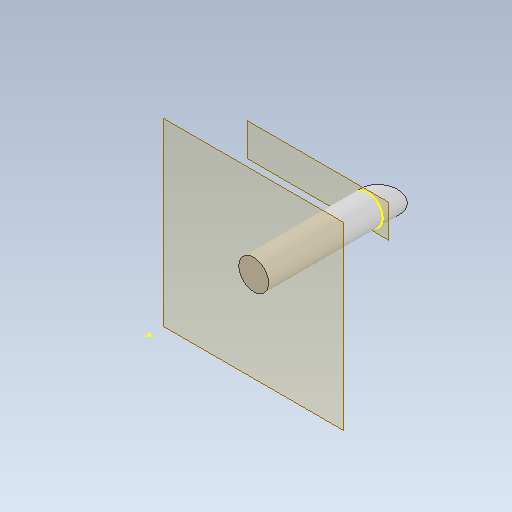
# Autodesk Inventor part: notch piston
Saved by Autodesk Inventor 2021 (Build 250183000, 183)
## iProperties
Created: 2021-03-12
Part Number: notch piston
Material: Generic
Document SubType Name: Modeling
Designer: teh18
Density: 1 g/cm^3
Appearance: Default
Author: teh18
Autodesk Inventor part; units mm, degrees
ref_plane "YZ Plane" through (0, 0, 0) normal (1, 0, 0) x (0, 1, 0)
ref_plane "XZ Plane" through (0, 0, 0) normal (0, 1, 0) x (-1, 0, 0)
sketch "Sketch1" plane through (0, 0, 0) normal (0, 0, 1) x (1, 0, 0)
  point P0 (0, 0)
ref_plane "Work Plane1" through (0, 0, -35) normal (0, 0, 1) x (1, 0, 0)
sketch "Sketch2" plane through (0, 0, -35) normal (0, 0, 1) x (1, 0, 0)
  circle A0 centre (0, 0) radius 5
  dimension "d0" = 10
  constraints: 1 centre point, 1 coincident
  measures "d0" diameter of A0
ref_plane "Work Plane2" through (46.1021, -24.8658, -116.0377) normal (0.6428, 0, 0.766) x (0.766, 0, -0.6428)
extrude "Extrusion1" add sketch "Sketch2" against normal up to surface surface through (46.1021, -24.8658, -116.0377) normal (0.6428, 0, 0.766)
ref_plane "Work Plane3" through (-5, 0, -73.1579) normal (0, 0, 1) x (1, 0, 0)
sketch "Sketch5" plane through (-5, 0, -73.1579) normal (0, 0, 1) x (1, 0, 0)
  circle A0 centre (5, 0) radius 5 projected
  point P0 (5, 0)
body "Solid1"
